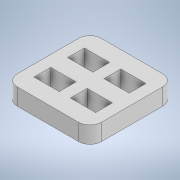
# Autodesk Inventor part: horn_base
Saved by Autodesk Inventor 2020 (Build 240168000, 168)
## iProperties
Created: 2020-07-26
Part Number: horn_base
Material: Generic
Document SubType Name: Modeling
Designer: Aarya
Density: 1 g/cm^3
Appearance: Default
Author: Aarya
Autodesk Inventor part; units mm, degrees
ref_plane "YZ Plane" through (0, 0, 0) normal (1, 0, 0) x (0, 1, 0)
ref_plane "XZ Plane" through (0, 0, 0) normal (0, 1, 0) x (-1, 0, 0)
ref_plane "XY Plane" through (0, 0, 0) normal (0, 0, 1) x (1, 0, 0)
sketch "Sketch1" plane through (0, 0, 0) normal (0, 1, 0) x (-1, 0, 0)
  line L0 (5.5, 7.5) -> (-5.5, 7.5)
  line L1 (-7.5, 5.5) -> (-7.5, -5.5)
  line L2 (-5.5, -7.5) -> (5.5, -7.5)
  line L3 (7.5, -5.5) -> (7.5, 5.5)
  line L4 (7.5, 7.5) -> (-7.5, -7.5) construction
  line L5 (-7.5, 7.5) -> (7.5, -7.5) construction
  arc A0 (7.5, 5.5) -> (5.5, 7.5) centre (5.5, 5.5) ccw
  arc A1 (-5.5, 7.5) -> (-7.5, 5.5) centre (-5.5, 5.5) ccw
  arc A2 (-7.5, -5.5) -> (-5.5, -7.5) centre (-5.5, -5.5) ccw
  arc A3 (5.5, -7.5) -> (7.5, -5.5) centre (5.5, -5.5) ccw
  line L6 (5.5, 4.5) -> (1, 4.5)
  line L7 (1, 4.5) -> (1, 1.5)
  line L8 (1, 1.5) -> (5.5, 1.5)
  line L9 (5.5, 1.5) -> (5.5, 4.5)
  line L10 (3.25, 0) -> (5.1677, 0)
  line L11 (0, 3.1331) -> (0, 1.6822) construction
  line L12 (5.5, -4.5) -> (1, -4.5)
  line L13 (1, -4.5) -> (1, -1.5)
  line L14 (1, -1.5) -> (5.5, -1.5)
  line L15 (5.5, -1.5) -> (5.5, -4.5)
  line L16 (-5.5, 4.5) -> (-1, 4.5)
  line L17 (-1, 4.5) -> (-1, 1.5)
  line L18 (-1, 1.5) -> (-5.5, 1.5)
  line L19 (-5.5, 1.5) -> (-5.5, 4.5)
  line L20 (-1, -4.5) -> (-1, -1.5)
  line L21 (-1, -1.5) -> (-5.5, -1.5)
  line L22 (-5.5, -1.5) -> (-5.5, -4.5)
  line L23 (-5.5, -4.5) -> (-1, -4.5)
  point P0 (0, 0)
  point P1 (5.5, -5.5)
  dimension "d0" = 2
  dimension "d1" = 11
  dimension "d2" = 11
  dimension "d5" = 3
  dimension "d6" = 4.5
  dimension "d7" = 2
  dimension "d8" = 3
  constraints: 48 end point, 13 symmetric about line, 8 point on circle, 8 point on line, 8 tangent, 4 centre point, 4 parallel, 3 equal radius, 2 horizontal, 2 midpoint, 2 perpendicular
  measures "d0" radius of A0
  measures "d1" distance of L2.start L2.end
  measures "d2" distance of L3.start L3.end
  measures "d5" distance of L8.end L6.start
  measures "d6" distance of L6.start L6.end
  measures "d7" distance between parallel lines of L9 L3
  measures "d8" distance between parallel lines of L6 L0
extrude "Extrusion1" add sketch "Sketch1" along normal blind 3
body "Solid1"
